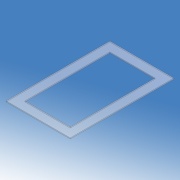
# Autodesk Inventor part: NASA-20-EBOX-T2-01
Saved by Autodesk Inventor 2020 (Build 240168000, 168)
## iProperties
Created: 2019-09-23
Part Number: NASA-20-EBOX-T2-01
Material: Polycarbonate, Clear
Document SubType Name: Modeling
Designer: mpark
Density: 1.2 g/cm^3
Appearance: Polycarbonate - Clear
Author: mpark
Autodesk Inventor part; units mm, degrees
ref_plane "YZ Plane" through (0, 0, 0) normal (1, 0, 0) x (0, 1, 0)
ref_plane "XZ Plane" through (0, 0, 0) normal (0, 1, 0) x (-1, 0, 0)
ref_plane "XY Plane" through (0, 0, 0) normal (0, 0, 1) x (1, 0, 0)
sketch "Sketch1" plane through (0, 0, 0) normal (0, 1, 0) x (-1, 0, 0)
  line L0 (107.95, -174.625) -> (-107.95, -174.625)
  line L1 (-107.95, -174.625) -> (-107.95, 174.625)
  line L2 (-107.95, 174.625) -> (107.95, 174.625)
  line L3 (107.95, 174.625) -> (107.95, -174.625)
  line L4 (107.95, -174.625) -> (-107.95, 174.625) construction
  line L5 (-107.95, -174.625) -> (107.95, 174.625) construction
  point P0 (0, 0)
  dimension "d0" = 215.9
  dimension "d1" = 349.25
  constraints: 12 end point, 2 midpoint, 2 parallel, 1 horizontal, 1 perpendicular
  measures "d0" distance of L1.end L2.end
  measures "d1" distance of L0.end L1.end
extrude "Thickness" add sketch "Sketch1" along normal blind 3.175
sketch "Cutout Sketch" plane through (0, 3.175, 0) normal (0, 1, 0) x (1, 0, 0)
  line L0 (107.95, -174.625) -> (107.95, 174.625) projected
  line L1 (107.95, 174.625) -> (-107.95, 174.625) projected
  line L2 (-107.95, 174.625) -> (-107.95, -174.625) projected
  line L3 (-107.95, -174.625) -> (107.95, -174.625) projected
  line L4 (-76.2, 142.875) -> (76.2, 142.875)
  line L5 (76.2, 142.875) -> (76.2, -142.875)
  line L6 (76.2, -142.875) -> (-76.2, -142.875)
  line L7 (-76.2, -142.875) -> (-76.2, 142.875)
  line L8 (-76.2, 142.875) -> (76.2, -142.875) construction
  line L9 (76.2, 142.875) -> (-76.2, -142.875) construction
  point P0 (0, 0)
  dimension "d4" = 31.75
  dimension "d5" = 31.75
  constraints: 12 end point, 2 midpoint, 2 parallel, 1 horizontal, 1 perpendicular
  measures "d4" distance between parallel lines of L7 L2
  measures "d5" distance between parallel lines of L1 L4
extrude "Cutout" cut sketch "Cutout Sketch" against normal blind 25.4 contours L4 L5 L6 L7
body "Solid1"
